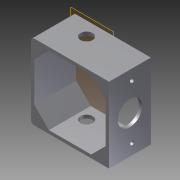
# Autodesk Inventor part: MotorHousingBottom_split3
Saved by Autodesk Inventor 2012 (Build 160160000, 160)
## iProperties
Created: 2011-12-19
Part Number: MotorHousingBottom_split3
Material: Default
Document SubType Name: Modeling
Designer: Drew
Density: 1 g/cm^3
Author: Drew
Autodesk Inventor part; units mm, degrees
ref_plane "YZ Plane" through (0, 0, 0) normal (1, 0, 0) x (0, 1, 0)
ref_plane "XZ Plane" through (0, 0, 0) normal (0, 1, 0) x (-1, 0, 0)
ref_plane "XY Plane" through (0, 0, 0) normal (0, 0, 1) x (1, 0, 0)
ref_plane "Work Plane1" through (0, 0, 0) normal (0, 0, 1) x (1, 0, 0)
sketch "Sketch3" plane through (0, 0, 0) normal (0, 0, 1) x (1, 0, 0)
  line L0 (-22.0216, 21.1569) -> (-22.0216, -21.1431) projected
  line L1 (-0.0216, 21.1569) -> (-22.0216, 21.1569) projected
  line L2 (-0.0216, 23.1569) -> (-0.0216, 21.1569) projected
  line L3 (-0.0216, 23.1569) -> (-22.0216, 23.1569) projected
  arc A0 (-22.0216, 23.1569) -> (-24.0216, 21.1569) centre (-22.0216, 21.1569) ccw projected
  line L4 (-24.0216, -21.1431) -> (-24.0216, 21.1569) projected
  arc A1 (-24.0216, -21.1431) -> (-22.0216, -23.1431) centre (-22.0216, -21.1431) ccw projected
  line L5 (-22.0216, -23.1431) -> (-0.0216, -23.1431) projected
  line L6 (-0.0216, -21.1431) -> (-0.0216, -23.1431) projected
  line L7 (-22.0216, -21.1431) -> (-0.0216, -21.1431) projected
  line L8 (0.2784, 23.1569) -> (0.2784, 21.1569) projected
  line L9 (12.9784, 21.1569) -> (0.2784, 21.1569) projected
  line L10 (21.9784, 12.1569) -> (12.9784, 21.1569) projected
  line L11 (21.9784, -12.1431) -> (21.9784, 12.1569) projected
  line L12 (12.9784, -21.1431) -> (21.9784, -12.1431) projected
  line L13 (0.2784, -21.1431) -> (12.9784, -21.1431) projected
  line L14 (0.2784, -21.1431) -> (0.2784, -23.1431) projected
  line L15 (23.9784, -23.1431) -> (0.2784, -23.1431) projected
  line L16 (23.9784, 23.1569) -> (23.9784, -23.1431) projected
  line L17 (0.2784, 23.1569) -> (23.9784, 23.1569) projected
  line L18 (0.2784, 21.1569) -> (-0.0216, 21.1569)
  line L19 (-0.0216, 21.1569) -> (-0.0216, 23.1569)
  line L20 (-0.0216, 23.1569) -> (0.2784, 23.1569)
  line L21 (0.2784, 23.1569) -> (0.2784, 21.1569)
  line L22 (-0.0216, -21.1431) -> (0.2784, -21.1431)
  line L23 (0.2784, -21.1431) -> (0.2784, -23.1431)
  line L24 (0.2784, -23.1431) -> (-0.0216, -23.1431)
  line L25 (-0.0216, -23.1431) -> (-0.0216, -21.1431)
  point P0 (0, 0)
  constraints: 16 end point, 4 parallel, 2 horizontal, 2 perpendicular
extrude "Extrusion2" add sketch "Sketch3" along normal blind 25.75 contours L0 L7 L6 L5 A1 L4 A0 L3 L2 L1 | L2 L20 L8 L18 | L22 L14 L24 L6 | L8 L17 L16 L15 L14 L13 L12 L11 L10 L9
sketch "Sketch5" plane through (23.9784, -23.1431, 0) normal (1, 0, 0) x (0, 0, -1)
  circle A0 centre (-12.875, 23.1431) radius 7.5
  point P0 (0, 23.1431)
  dimension "d4" = 15
  constraints: 1 centre point
  measures "d4" diameter of A0
extrude "Extrusion3" cut sketch "Sketch5" against normal up to surface (2 mm away)
sketch "Sketch6" plane through (-22.0216, -23.1431, 0) normal (0, -1, 0) x (1, 0, 0)
  circle A0 centre (15, 8.5833) radius 3.75
  line L0 (46, 25.75) -> (0, 25.75) projected
  line L1 (0, 0) -> (0, 25.75) projected
  point P0 (22.0216, 0)
  dimension "d7" = 7.5
  dimension "d10" = 25.75
  dimension "d11" = 17.1667
  dimension "d12" = 15
  constraints: 1 centre point
  measures "d7" diameter of A0
  measures "d10" distance of L1.start L0.end
  measures "d11" distance from line of L0 A0.centre
  measures "d12" distance from line of L1 A0.centre
extrude "Extrusion4" cut sketch "Sketch6" against normal through all
sketch "Sketch7" plane through (0, 0, 25.75) normal (0, 0, 1) x (1, 0, 0)
  line L0 (-22.0216, -21.1431) -> (12.9784, -21.1431) projected
  line L1 (-22.0216, 21.1569) -> (-22.0216, -21.1431) projected
  line L2 (-22.0216, -12.1431) -> (-22.0216, -21.1431) projected
  line L3 (-22.0216, -12.1431) -> (-13.0216, -21.1431) projected
  line L4 (-22.0216, -21.1431) -> (-13.0216, -21.1431) projected
  line L5 (-13.0216, 21.1569) -> (-22.0216, 21.1569) projected
  line L6 (-13.0216, 21.1569) -> (-22.0216, 12.1569) projected
  line L7 (-22.0216, 21.1569) -> (-22.0216, 12.1569) projected
  point P0 (0, 0)
ref_plane "Work Plane2" through (-24.0216, -23.1431, 0) normal (0, 0, 1) x (1, 0, 0)
extrude "Extrusion5" add sketch "Sketch7" against normal up to surface (25.75 mm away)
sketch "Sketch8" plane through (23.9784, -23.1431, 0) normal (1, 0, 0) x (0, 0, -1)
  circle A0 centre (-11.625, 39.8) radius 1.25 projected
  circle A1 centre (-11.625, 6.5) radius 1.25 projected
  point P0 (0, 23.1431)
extrude "Extrusion6" cut sketch "Sketch8" against normal blind 25.75
equation "\"d11\" = 0.666667 * d10"
body "Solid2"
